Autodesk Inventor part; units mm, degrees
(part 3 of 3)
  arc A490 (-2990.6524, -2157.8219) -> (-2908.1943, -2279.9148) centre (-1432.224, -1194.1948) ccw
  arc A491 (-2908.1943, -2279.9148) -> (-2818.7411, -2390.8385) centre (-1616.1239, -1329.4704) ccw
  arc A492 (-2779.4113, -2436.604) -> (-2818.7411, -2390.8385) centre (-4535.4377, -3905.9087) ccw
  arc A493 (-2757.2128, -2466.1631) -> (-2779.4113, -2436.604) centre (-3049.0332, -2662.2024) ccw
  arc A494 (-2745.8364, -2486.6243) -> (-2757.2128, -2466.1631) centre (-2872.8883, -2543.8714) ccw
  arc A495 (-2745.9498, -2499.1945) -> (-2745.8364, -2486.6243) centre (-2759.5126, -2492.7865) ccw
  arc A496 (-2745.9498, -2499.1945) -> (-2749.3057, -2511.7301) centre (-2713.1452, -2514.6935) ccw
  arc A497 (-2749.3057, -2511.7301) -> (-2753.148, -2562.4823) centre (1336.3779, -2846.57) ccw
  arc A498 (-2753.148, -2562.4823) -> (-2756.6405, -2622.7286) centre (-124.1368, -2745.1096) ccw
  arc A499 (-2756.6405, -2622.7286) -> (-2759.272, -2690.9741) centre (1553.6701, -2823.1066) ccw
  line L62 (-2759.272, -2690.9741) -> (-2764.631, -2865.8991)
  line L63 (-2764.631, -2865.8991) -> (-2835.8911, -2780.9741)
  arc A500 (-2918.8006, -2674.4171) -> (-2835.8911, -2780.9741) centre (-1434.1321, -1604.7647) ccw
  arc A501 (-2986.2074, -2570.7172) -> (-2918.8006, -2674.4171) centre (-1871.837, -1920.1137) ccw
  arc A502 (-3041.5026, -2464.1872) -> (-2986.2074, -2570.7172) centre (-1942.3549, -1961.2823) ccw
  arc A503 (-3087.9821, -2349.1865) -> (-3041.5026, -2464.1872) centre (-1788.2283, -1890.7618) ccw
  arc A504 (-3121.0778, -2239.9227) -> (-3087.9821, -2349.1865) centre (-1890.4003, -1926.7975) ccw
  arc A505 (-3139.0551, -2142.0083) -> (-3121.0778, -2239.9227) centre (-2406.5893, -2058.1334) ccw
  arc A506 (-3147.4064, -2018.8391) -> (-3139.0551, -2142.0083) centre (-1814.454, -1990.3279) ccw
  arc A507 (-3149.631, -1810.813) -> (-3147.4064, -2018.8391) centre (6577.4997, -1810.8179) ccw
  line L64 (-3149.631, -1810.813) -> (-3149.631, -1522.7863)
  line L65 (-3149.631, -1522.7863) -> (-3120.6403, -1533.7291)
  arc A508 (-3120.6403, -1533.7291) -> (-3104.6551, -1538.5038) centre (-3078.921, -1423.2019) ccw
  arc A509 (-3104.6551, -1538.5038) -> (-3092.2345, -1539.1823) centre (-3096.4076, -1501.5506) ccw
  arc A510 (-3092.2345, -1539.1823) -> (-3080.2478, -1535.7989) centre (-3096.4218, -1501.4224) ccw
  arc A511 (-3080.2478, -1535.7989) -> (-3065.6403, -1527.6299) centre (-3131.0839, -1427.7506) ccw
  line L66 (-3065.6403, -1527.6299) -> (-3039.631, -1510.588)
  line L67 (-3039.631, -1510.588) -> (-3039.631, -70.8185)
  arc A512 (-3039.3783, 481.2624) -> (-3039.631, -70.8185) centre (599668.8589, -70.706) ccw
  arc A513 (-3038.5978, 946.0187) -> (-3039.3783, 481.2624) centre (301120.8498, 202.8683) ccw
  arc A514 (-3036.1137, 1368.9509) -> (-3037.5632, 1367.505) centre (-3036.1137, 1367.5015) ccw
  arc A515 (-3033.5939, 1368.2338) -> (-3036.1137, 1368.9509) centre (-3036.1137, 1364.1654) ccw
  arc A516 (-3013.7437, 1355.8898) -> (-3033.5939, 1368.2338) centre (-6444.9521, -4139.6549) ccw
  arc A517 (-2991.1032, 1341.5314) -> (-3013.7437, 1355.8898) centre (-4021.8968, -258.8014) ccw
  arc A518 (-2964.8997, 1324.4876) -> (-2991.1032, 1341.5314) centre (-4889.5902, -1605.9104) ccw
  arc A519 (3062.8013, -60.9811) -> (3061.4495, -1006.9802) centre (1295410.6067, -2380.7565) ccw
  arc A520 (3061.4495, -1006.9802) -> (3063.1224, -1310.9835) centre (26211.8445, -1031.5883) ccw
  arc A521 (3063.1224, -1310.9835) -> (3066.6099, -1479.2538) centre (12786.7982, -1193.6248) ccw
  arc A522 (3066.6099, -1479.2538) -> (3080.3013, -1510.9814) centre (3113.4039, -1477.8788) ccw
  arc A523 (3080.3013, -1510.9814) -> (3097.9046, -1523.8965) centre (3131.1382, -1460.1446) ccw
  arc A524 (3097.9046, -1523.8965) -> (3117.6763, -1530.0742) centre (3124.9899, -1471.939) ccw
  arc A525 (3117.6763, -1530.0742) -> (3138.8082, -1529.0661) centre (3125.3546, -1469.0395) ccw
  arc A526 (3138.8082, -1529.0661) -> (3160.3613, -1521.0532) centre (3120.1885, -1445.9896) ccw
  arc A527 (3170.8286, -1524.3232) -> (3160.3613, -1521.0532) centre (3163.9885, -1527.8306) ccw
  arc A528 (3176.5518, -1544.1089) -> (3170.8286, -1524.3232) centre (3122.861, -1548.9189) ccw
  arc A529 (3178.9628, -1593.2927) -> (3176.5518, -1544.1089) centre (2568.873, -1598.5484) ccw
  arc A530 (3179.8463, -1738.5532) -> (3178.9628, -1593.2927) centre (-25505.4744, -1840.3836) ccw
  arc A531 (3175.9829, -1976.8584) -> (3179.8463, -1738.5532) centre (-2851.4872, -1759.9572) ccw
  arc A532 (3160.8237, -2144.1805) -> (3175.9829, -1976.8584) centre (1631.4842, -1921.2765) ccw
  arc A533 (3130.6102, -2282.5675) -> (3160.8237, -2144.1805) centre (2161.9433, -1998.5905) ccw
  arc A534 (3079.9973, -2423.6115) -> (3130.6102, -2282.5675) centre (1918.6719, -1927.2727) ccw
  arc A535 (3039.5585, -2510.0751) -> (3079.9973, -2423.6115) centre (1772.8663, -1864.9587) ccw
  arc A536 (2995.4615, -2588.7548) -> (3039.5585, -2510.0751) centre (2029.2646, -1995.5405) ccw
  arc A537 (2943.0501, -2667.3464) -> (2995.4615, -2588.7548) centre (1922.5744, -1930.036) ccw
  arc A538 (2877.3135, -2753.7324) -> (2943.0501, -2667.3464) centre (1169.0771, -1385.6217) ccw
  line L68 (2877.3135, -2753.7324) -> (2795.369, -2856.0491)
  line L69 (2795.369, -2856.0491) -> (2789.4968, -2696.0491)
  arc A539 (2789.4968, -2696.0491) -> (2786.3804, -2632.67) centre (242.2861, -2789.5322) ccw
  arc A540 (2786.3804, -2632.67) -> (2781.8611, -2574.5881) centre (977.5322, -2744.1986) ccw
  arc A541 (2781.8611, -2574.5881) -> (2776.6989, -2526.2333) centre (864.468, -2754.8287) ccw
  arc A542 (2776.6989, -2526.2333) -> (2771.7488, -2507.2457) centre (2704.8711, -2534.82) ccw
  arc A543 (2767.4869, -2488.0525) -> (2771.7488, -2507.2457) centre (2824.6766, -2485.4232) ccw
  arc A544 (2771.2401, -2471.7334) -> (2767.4869, -2488.0525) centre (2798.6183, -2486.6212) ccw
  arc A545 (2786.0079, -2450.4453) -> (2771.2401, -2471.7334) centre (2876.4028, -2528.9192) ccw
  arc A546 (2829.1062, -2401.7678) -> (2786.0079, -2450.4453) centre (5301.222, -4633.9592) ccw
  arc A547 (2829.1062, -2401.7678) -> (2920.7467, -2290.528) centre (1649.3147, -1336.4763) ccw
  arc A548 (2920.7467, -2290.528) -> (3006.9234, -2165.8357) centre (1366.1527, -1123.9981) ccw
  arc A549 (3006.9234, -2165.8357) -> (3074.9751, -2050.5252) centre (1272.0921, -1064.2721) ccw
  arc A550 (3074.9751, -2050.5252) -> (3090.369, -1990.3095) centre (2964.9004, -1990.3095) ccw
  arc A551 (3090.369, -1990.3095) -> (3086.1599, -1969.8686) centre (3038.6292, -1990.3096) ccw
  arc A552 (3086.1599, -1969.8686) -> (3073.9361, -1950.2444) centre (3015.5336, -2000.2421) ccw
  arc A553 (3073.9361, -1950.2444) -> (3057.1368, -1935.9564) centre (3020.6955, -1995.8229) ccw
  arc A554 (3057.1368, -1935.9564) -> (3039.637, -1931.0491) centre (3039.637, -1964.7055) ccw
  arc A555 (3039.637, -1931.0491) -> (3014.6452, -1935.8643) centre (3039.637, -1998.3124) ccw
  arc A556 (3014.6452, -1935.8643) -> (2994.6509, -1949.5434) centre (3035.33, -1987.5505) ccw
  arc A557 (2994.6509, -1949.5434) -> (2973.9887, -1977.5702) centre (3104.4016, -2052.0851) ccw
  arc A558 (2973.9887, -1977.5702) -> (2943.1237, -2034.3477) centre (4298.6367, -2734.4439) ccw
  arc A559 (2902.337, -2106.6921) -> (2943.1237, -2034.3477) centre (1935.3983, -1513.8772) ccw
  arc A560 (2855.8027, -2176.9427) -> (2902.337, -2106.6921) centre (1877.629, -1478.4583) ccw
  arc A561 (2802.0044, -2247.2249) -> (2855.8027, -2176.9427) centre (1771.3658, -1402.5793) ccw
  arc A562 (2739.3728, -2319.6849) -> (2802.0044, -2247.2249) centre (1389.8938, -1089.9508) ccw
  line L70 (2739.3728, -2319.6849) -> (2683.3767, -2381.1337)
  line L71 (2683.3767, -2381.1337) -> (2632.1085, -2358.5914)
  line L72 (2632.1085, -2358.5914) -> (2580.8403, -2336.0491)
  line L73 (2580.8403, -2336.0491) -> (2580.6421, -711.0491)
  line L74 (2580.6421, -711.0491) -> (2580.4439, 913.9509)
  line L75 (2580.4439, 913.9509) -> (2623.3363, 931.5853)
  arc A563 (2623.3363, 931.5853) -> (2684.605, 968.0874) centre (2530.9143, 1156.3857) ccw
  arc A564 (2684.605, 968.0874) -> (2734.8197, 1021.8078) centre (2511.3163, 1180.3966) ccw
  arc A565 (2734.8197, 1021.8078) -> (2770.0399, 1088.4458) centre (2499.3492, 1188.8877) ccw
  arc A566 (2770.0399, 1088.4458) -> (2787.3675, 1162.7589) centre (2485.9178, 1193.8713) ccw
  arc A567 (2792.105, 1195.7029) -> (2787.3675, 1162.7589) centre (3201.5168, 1120.0149) ccw
  arc A568 (2799.1005, 1211.8828) -> (2792.105, 1195.7029) centre (2830.904, 1188.5302) ccw
  arc A569 (2812.8006, 1224.3388) -> (2799.1005, 1211.8828) centre (2836.7429, 1184.2428) ccw
  arc A570 (2846.3908, 1243.1416) -> (2812.8006, 1224.3388) centre (3165.391, 633.8599) ccw
  arc A571 (2846.3908, 1243.1416) -> (2872.3676, 1257.2794) centre (2420.1812, 2057.1904) ccw
  arc A572 (2872.3676, 1257.2794) -> (2907.0809, 1277.2085) centre (1391.313, 3877.2384) ccw
  arc A573 (2907.0809, 1277.2085) -> (2944.0271, 1299.0743) centre (1263.5319, 4096.4282) ccw
  arc A574 (2944.0271, 1299.0743) -> (2977.6923, 1319.6879) centre (1742.0091, 3299.9558) ccw
  arc A575 (3007.8259, 1338.2944) -> (2977.6923, 1319.6879) centre (4966.2802, -1867.1663) ccw
  arc A576 (3034.0202, 1354.0365) -> (3007.8259, 1338.2944) centre (4097.0708, -444.5093) ccw
  arc A577 (3056.8159, 1367.4393) -> (3034.0202, 1354.0365) centre (5954.021, -3586.2434) ccw
  arc A578 (3060.369, 1368.5548) -> (3056.8159, 1367.4393) centre (3061.0292, 1360.2354) ccw
  arc A579 (3062.4249, 1366.6589) -> (3060.369, 1368.5548) centre (3060.5197, 1366.6556) ccw
  arc A580 (3063.146, 948.7923) -> (3062.4249, 1366.6589) centre (-8702491.5883, -13865.3994) ccw
  arc A581 (3063.4266, 487.3009) -> (3063.146, 948.7923) centre (-207855.965, 589.788) ccw
  arc A582 (3062.8013, -60.9811) -> (3063.4266, 487.3009) centre (-414834.6536, 689.7528) ccw
  arc A583 (-1913.5687, 954.2396) -> (-1734.4782, 921.0323) centre (-866.4512, 6101.9309) ccw
  arc A584 (-1734.4782, 921.0323) -> (-1529.2527, 889.1161) centre (-270.2991, 9660.1238) ccw
  arc A585 (-1529.2527, 889.1161) -> (-1316.4625, 861.0585) centre (-198.9574, 10157.2039) ccw
  arc A586 (-1316.4625, 861.0585) -> (-1114.075, 839.4841) centre (-412.5654, 8380.3495) ccw
  arc A587 (-1114.075, 839.4841) -> (-975.393, 827.6361) centre (-258.4444, 10037.1738) ccw
  arc A588 (-975.393, 827.6361) -> (-837.5262, 817.9702) centre (-278.4862, 9779.7099) ccw
  arc A589 (-837.5262, 817.9702) -> (-657.2277, 807.634) centre (279.2554, 18720.7697) ccw
  arc A590 (-657.2277, 807.634) -> (-362.1635, 792.5791) centre (5502.6263, 118637.185) ccw
  line L76 (-362.1635, 792.5791) -> (-249.696, 786.982)
  line L77 (-249.696, 786.982) -> (-230.6402, 743.9032)
  arc A591 (-230.6402, 743.9032) -> (-205.8315, 701.8713) centre (-39.0236, 828.6645) ccw
  arc A592 (-205.8315, 701.8713) -> (-168.5998, 660.0881) centre (80.3764, 919.4226) ccw
  arc A593 (-168.5998, 660.0881) -> (-126.8329, 625.9013) centre (67.9455, 906.4746) ccw
  arc A594 (-126.8329, 625.9013) -> (-88.4851, 607.4261) centre (-49.6317, 737.1074) ccw
  line L78 (-88.4851, 607.4261) -> (-49.631, 595.7852)
  line L79 (-49.631, 595.7852) -> (-49.631, -1176.8374)
  line L80 (-49.631, -1176.8374) -> (-49.631, -2949.46)
  line L81 (-49.631, -2949.46) -> (-79.3693, -2955.9916)
  arc A595 (-79.3693, -2955.9916) -> (-115.6838, -2972.2525) centre (-58.3842, -3051.5361) ccw
  arc A596 (-115.6838, -2972.2525) -> (-160.8987, -3009.8378) centre (138.8628, -3324.4606) ccw
  arc A597 (-160.8987, -3009.8378) -> (-201.9746, -3054.7507) centre (144.5508, -3330.4312) ccw
  arc A598 (-201.9746, -3054.7507) -> (-226.1643, -3095.8525) centre (-68.3247, -3161.077) ccw
  line L82 (-226.1643, -3095.8525) -> (-244.631, -3140.541)
  line L83 (-244.631, -3140.541) -> (-349.631, -3135.1711)
  arc A599 (-882.8658, -3087.8365) -> (-349.631, -3135.1711) centre (15.6016, 4006.431) ccw
  arc A600 (-1366.8413, -3002.6041) -> (-882.8658, -3087.8365) centre (-244.0669, 1956.1506) ccw
  arc A601 (-1799.9599, -2880.1482) -> (-1366.8413, -3002.6041) centre (-426.4321, 1150.7475) ccw
  arc A602 (-2180.0572, -2720.7229) -> (-1799.9599, -2880.1482) centre (-832.1243, -39.841) ccw
  line L84 (-2180.0572, -2720.7229) -> (-2235.4834, -2692.8549)
  line L85 (-2235.4834, -2692.8549) -> (-2237.9929, -2610.9162)
  arc A603 (-2237.9929, -2610.9162) -> (-2240.3199, -2571.0685) centre (-2957.8229, -2632.9615) ccw
  arc A604 (-2240.3199, -2571.0685) -> (-2244.7516, -2538.0792) centre (-2589.6104, -2601.1989) ccw
  arc A605 (-2244.7516, -2538.0792) -> (-2251.5187, -2510.0686) centre (-2497.873, -2584.4084) ccw
  arc A606 (-2251.5187, -2510.0686) -> (-2260.9536, -2485.4694) centre (-2424.0386, -2562.1284) ccw
  arc A607 (-2260.9536, -2485.4694) -> (-2285.6695, -2445.4611) centre (-2448.0589, -2573.4192) ccw
  arc A608 (-2285.6695, -2445.4611) -> (-2322.761, -2404.7458) centre (-2588.4779, -2684.0657) ccw
  arc A609 (-2322.761, -2404.7458) -> (-2364.4619, -2370.44) centre (-2581.3125, -2676.5338) ccw
  arc A610 (-2364.4619, -2370.44) -> (-2403.1079, -2350.2383) centre (-2458.3199, -2502.9245) ccw
  line L86 (-2403.1079, -2350.2383) -> (-2439.631, -2337.0313)
  line L87 (-2439.631, -2337.0313) -> (-2439.5936, -711.5402)
  line L88 (-2439.5936, -711.5402) -> (-2439.5561, 913.9509)
  line L89 (-2439.5561, 913.9509) -> (-2396.4619, 931.6687)
  arc A611 (-2396.4619, 931.6687) -> (-2376.9013, 941.5424) centre (-2450.351, 1062.7406) ccw
  arc A612 (-2376.9013, 941.5424) -> (-2353.4806, 956.9654) centre (-2570.7261, 1261.3703) ccw
  arc A613 (-2353.4806, 956.9654) -> (-2330.1607, 974.9443) centre (-2585.0508, 1281.4419) ccw
  arc A614 (-2330.1607, 974.9443) -> (-2310.6579, 992.9047) centre (-2498.0086, 1176.7758) ccw
  line L90 (-2310.6579, 992.9047) -> (-2267.9481, 1036.4228)
  line L91 (-2267.9481, 1036.4228) -> (-2176.2896, 1012.7295)
  arc A615 (-2176.2896, 1012.7295) -> (-2129.5346, 1001.2725) centre (-1700.0863, 2854.9472) ccw
  arc A616 (-2129.5346, 1001.2725) -> (-2061.3062, 985.7746) centre (-293.3415, 8927.0311) ccw
  arc A617 (-2061.3062, 985.7746) -> (-1985.782, 969.299) centre (-96.1324, 9812.7982) ccw
  arc A618 (-1985.782, 969.299) -> (-1913.5687, 954.2396) centre (-418.6364, 8303.4593) ccw
  arc A619 (2330.7457, 994.7005) -> (2349.6048, 976.4208) centre (2502.3822, 1152.9096) ccw
  arc A620 (2349.6048, 976.4208) -> (2372.5893, 958.0878) centre (2588.9145, 1252.8727) ccw
  arc A621 (2372.5893, 958.0878) -> (2395.987, 942.3436) centre (2577.2368, 1236.9605) ccw
  arc A622 (2395.987, 942.3436) -> (2415.9142, 932.2005) centre (2468.6632, 1060.4771) ccw
  line L92 (2415.9142, 932.2005) -> (2460.294, 913.9509)
  line L93 (2460.294, 913.9509) -> (2460.3315, -712.7545)
  line L94 (2460.3315, -712.7545) -> (2460.369, -2339.46)
  line L95 (2460.369, -2339.46) -> (2430.6307, -2345.9916)
  arc A623 (2430.6307, -2345.9916) -> (2395.6917, -2361.6356) centre (2450.823, -2437.9267) ccw
  arc A624 (2395.6917, -2361.6356) -> (2350.0869, -2399.0009) centre (2680.5345, -2755.8033) ccw
  arc A625 (2350.0869, -2399.0009) -> (2307.6277, -2443.56) centre (2685.108, -2760.7414) ccw
  arc A626 (2307.6277, -2443.56) -> (2281.1542, -2484.427) centre (2458.3519, -2570.2071) ccw
  arc A627 (2281.1542, -2484.427) -> (2271.1872, -2509.3607) centre (2452.5649, -2567.4054) ccw
  arc A628 (2271.1872, -2509.3607) -> (2264.8592, -2535.3799) centre (2450.5721, -2566.7676) ccw
  arc A629 (2264.8592, -2535.3799) -> (2261.4364, -2566.4384) centre (2532.1364, -2580.5531) ccw
  arc A630 (2261.4364, -2566.4384) -> (2260.369, -2607.4076) centre (3047.127, -2607.4068) ccw
  line L96 (2260.369, -2607.4076) -> (2260.369, -2687.4517)
  line L97 (2260.369, -2687.4517) -> (2157.869, -2738.3674)
  arc A631 (1885.6632, -2855.5638) -> (2157.869, -2738.3674) centre (947.2098, -301.1524) ccw
  arc A632 (1576.3744, -2954.8591) -> (1885.6632, -2855.5638) centre (533.2985, 825.4938) ccw
  arc A633 (1238.9166, -3033.9584) -> (1576.3744, -2954.8591) centre (393.5214, 1332.1036) ccw
  arc A634 (881.9152, -3090.4282) -> (1238.9166, -3033.9584) centre (239.5431, 2127.3587) ccw
  arc A635 (774.7121, -3102.6312) -> (881.9152, -3090.4282) centre (161.6389, 2760.1604) ccw
  arc A636 (664.968, -3113.1563) -> (774.7121, -3102.6312) centre (106.361, 3288.8229) ccw
  arc A637 (534.0943, -3123.6818) -> (664.968, -3113.1563) centre (-176.4478, 6530.0766) ccw
  arc A638 (358.5435, -3136.0948) -> (534.0943, -3123.6818) centre (-1710.2072, 27368.8116) ccw
  line L98 (358.5435, -3136.0948) -> (271.7179, -3141.9829)
  line L99 (271.7179, -3141.9829) -> (252.0201, -3097.4527)
  arc A639 (252.0201, -3097.4527) -> (226.8939, -3054.645) centre (53.0153, -3185.4819) ccw
  arc A640 (226.8939, -3054.645) -> (189.6185, -3012.4784) centre (-58.6317, -3269.4916) ccw
  arc A641 (189.6185, -3012.4784) -> (147.8207, -2978.1362) centre (-44.7457, -3255.1153) ccw
  arc A642 (147.8207, -2978.1362) -> (109.223, -2959.5243) centre (70.1942, -3089.7909) ccw
  line L100 (109.223, -2959.5243) -> (70.369, -2947.8833)
  line L101 (70.369, -2947.8833) -> (70.369, -1180.6397)
  line L102 (70.369, -1180.6397) -> (70.369, 586.6039)
  line L103 (70.369, 586.6039) -> (124.685, 613.1783)
  arc A643 (124.685, 613.1783) -> (167.8117, 638.9579) centre (-7.2831, 882.9109) ccw
  arc A644 (167.8117, 638.9579) -> (205.1584, 671.1351) centre (5.4675, 865.1457) ccw
  arc A645 (205.1584, 671.1351) -> (235.1633, 708.2885) centre (17.9614, 853.0072) ccw
  arc A646 (235.1633, 708.2885) -> (256.4939, 748.8465) centre (50.7207, 831.1804) ccw
  line L104 (256.4939, 748.8465) -> (271.8098, 787.1245)
  line L105 (271.8098, 787.1245) -> (373.5894, 792.4972)
  arc A647 (427.4041, 795.2935) -> (373.5894, 792.4972) centre (2101.4454, -31940.1076) ccw
  arc A648 (511.565, 799.578) -> (427.4041, 795.2935) centre (9783.5496, -182160.9748) ccw
  arc A649 (606.7619, 804.3802) -> (511.565, 799.578) centre (10908.7538, -204363.8155) ccw
  arc A650 (700.369, 809.0576) -> (606.7619, 804.3802) centre (10238.2989, -191011.0651) ccw
  arc A651 (700.369, 809.0576) -> (1093.0397, 836.3644) centre (205.3886, 10763.7794) ccw
  arc A652 (1093.0397, 836.3644) -> (1472.2395, 878.5747) centre (309.3592, 9601.0173) ccw
  arc A653 (1472.2395, 878.5747) -> (1822.03, 933.4564) centre (458.966, 8478.8527) ccw
  arc A654 (1822.03, 933.4564) -> (2125.369, 999.0389) centre (1015.3399, 5398.953) ccw
  arc A655 (2183.3894, 1013.6184) -> (2125.369, 999.0389) centre (9876.5597, -29724.835) ccw
  arc A656 (2233.4491, 1026.0693) -> (2183.3894, 1013.6184) centre (6454.9688, -16053.7077) ccw
  arc A657 (2277.1003, 1036.8395) -> (2233.4491, 1026.0693) centre (15584.8039, -52992.3058) ccw
  arc A658 (2282.663, 1037.9163) -> (2277.1003, 1036.8395) centre (2290.577, 982.1241) ccw
  arc A659 (2287.1065, 1036.6495) -> (2282.663, 1037.9163) centre (2283.4612, 1032.2895) ccw
  arc A660 (2299.7961, 1025.6484) -> (2287.1065, 1036.6495) centre (1986.1488, 676.6788) ccw
  arc A661 (2314.5869, 1011.582) -> (2299.7961, 1025.6484) centre (2057.4823, 756.0457) ccw
  arc A662 (2330.7457, 994.7005) -> (2314.5869, 1011.582) centre (1874.0627, 573.7448) ccw
  arc A663 (2490.9409, -2639.684) -> (2505.8853, -2646.7865) centre (2551.8525, -2530.7929) ccw
  arc A664 (2505.8853, -2646.7865) -> (2517.1948, -2648.9704) centre (2517.3254, -2617.9183) ccw
  arc A665 (2517.1948, -2648.9704) -> (2529.0128, -2646.9546) centre (2517.3411, -2614.177) ccw
  arc A666 (2529.0128, -2646.9546) -> (2545.9409, -2639.9153) centre (2469.8448, -2480.7932) ccw
  arc A667 (2545.9409, -2639.9153) -> (2563.237, -2628.9559) centre (2508.6457, -2561.9285) ccw
  arc A668 (2563.237, -2628.9559) -> (2571.7932, -2616.5764) centre (2546.1929, -2608.0291) ccw
  arc A669 (2571.7932, -2616.5764) -> (2575.7925, -2595.8507) centre (2495.5121, -2591.1081) ccw
  arc A670 (2575.7925, -2595.8507) -> (2578.2797, -2543.0571) centre (364.474, -2465.2187) ccw
  line L106 (2578.2797, -2543.0571) -> (2581.1904, -2460.2721)
  line L107 (2581.1904, -2460.2721) -> (2609.6423, -2480.5316)
  arc A671 (2643.4506, -2519.1082) -> (2609.6423, -2480.5316) centre (2545.0501, -2571.243) ccw
  arc A672 (2661.2042, -2573.3624) -> (2643.4506, -2519.1082) centre (2495.2127, -2597.6479) ccw
  arc A673 (2668.8278, -2669.1243) -> (2661.2042, -2573.3624) centre (1938.7489, -2679.0613) ccw
  arc A674 (2670.369, -2895.6004) -> (2668.8278, -2669.1243) centre (-13973.0742, -2895.6158) ccw
  arc A675 (2669.6986, -3030.0281) -> (2670.369, -2895.6004) centre (-10804.9877, -2895.6124) ccw
  arc A676 (2667.5603, -3134.2249) -> (2669.6986, -3030.0281) centre (-2272.2812, -2980.7323) ccw
  arc A677 (2664.4733, -3214.9061) -> (2667.5603, -3134.2249) centre (-2952.3801, -2959.5989) ccw
  arc A678 (2659.7328, -3237.8981) -> (2664.4733, -3214.9061) centre (2589.9098, -3211.5171) ccw
  arc A679 (2617.088, -3299.3064) -> (2659.7328, -3237.8981) centre (2515.9908, -3183.5884) ccw
  arc A680 (2550.958, -3332.4809) -> (2617.088, -3299.3064) centre (2519.8906, -3188.0521) ccw
  arc A681 (2477.58, -3329.2633) -> (2550.958, -3332.4809) centre (2520.4231, -3190.527) ccw
  arc A682 (2414.8927, -3290.5645) -> (2477.58, -3329.2633) centre (2520.9094, -3188.9526) ccw
  line L108 (2414.8927, -3290.5645) -> (2385.369, -3259.761)
  line L109 (2385.369, -3259.761) -> (2382.3531, -2922.905)
  arc A683 (2381.6256, -2791.5061) -> (2382.3531, -2922.905) centre (21614.7948, -2750.7158) ccw
  arc A684 (2381.9551, -2675.5679) -> (2381.6256, -2791.5061) centre (14059.6173, -2766.7308) ccw
  arc A685 (2382.9678, -2577.1763) -> (2381.9551, -2675.5679) centre (22171.5681, -2830.0363) ccw
  arc A686 (2385.2333, -2553.9382) -> (2382.9678, -2577.1763) centre (2521.4308, -2578.9456) ccw
  arc A687 (2389.7676, -2539.3341) -> (2385.2333, -2553.9382) centre (2448.3349, -2565.5244) ccw
  arc A688 (2398.8325, -2521.8027) -> (2389.7676, -2539.3341) centre (2548.7354, -2610.4216) ccw
  arc A689 (2410.5199, -2504.3143) -> (2398.8325, -2521.8027) centre (2562.8614, -2618.7725) ccw
  arc A690 (2423.2491, -2489.6327) -> (2410.5199, -2504.3143) centre (2521.6666, -2587.8218) ccw
  line L110 (2423.2491, -2489.6327) -> (2455.369, -2457.4382)
  line L111 (2455.369, -2457.4382) -> (2460.369, -2541.4088)
  arc A691 (2460.369, -2541.4088) -> (2464.0505, -2591.6371) centre (4296.3427, -2432.0873) ccw
  arc A692 (2464.0505, -2591.6371) -> (2468.5613, -2614.5688) centre (2572.6845, -2582.1776) ccw
  arc A693 (2468.5613, -2614.5688) -> (2476.6105, -2628.4384) centre (2502.9909, -2603.8582) ccw
  arc A694 (2476.6105, -2628.4384) -> (2490.9409, -2639.684) centre (2519.6793, -2588.3087) ccw
  arc A695 (-2559.631, -2541.0491) -> (-2556.1243, -2591.8911) centre (-2189.3068, -2541.0489) ccw
  arc A696 (-2556.1243, -2591.8911) -> (-2544.5669, -2625.2727) centre (-2466.0956, -2579.4128) ccw
  arc A697 (-2544.5669, -2625.2727) -> (-2524.4099, -2644.1736) centre (-2502.6649, -2600.7846) ccw
  arc A698 (-2524.4099, -2644.1736) -> (-2495.3453, -2651.0491) centre (-2495.3453, -2586.1796) ccw
  arc A699 (-2495.3453, -2651.0491) -> (-2468.5276, -2645.1415) centre (-2495.3453, -2587.2255) ccw
  arc A700 (-2468.5276, -2645.1415) -> (-2451.346, -2628.8207) centre (-2484.071, -2611.5738) ccw
  arc A701 (-2451.346, -2628.8207) -> (-2442.1698, -2598.1342) centre (-2524.6584, -2590.1831) ccw
  arc A702 (-2442.1698, -2598.1342) -> (-2439.631, -2545.3348) centre (-2989.9362, -2545.3347) ccw
  arc A703 (-2439.3304, -2516.8507) -> (-2439.631, -2545.3348) centre (-1090.074, -2545.3353) ccw
  arc A704 (-2438.4025, -2492.8705) -> (-2439.3304, -2516.8507) centre (-1756.3445, -2531.2692) ccw
  arc A705 (-2437.1381, -2472.6263) -> (-2438.4025, -2492.8705) centre (-788.7023, -2585.7452) ccw
  arc A706 (-2435.4489, -2471.0491) -> (-2437.1381, -2472.6263) centre (-2435.4489, -2472.7423) ccw
  arc A707 (-2421.7438, -2474.1426) -> (-2435.4489, -2471.0491) centre (-2435.4489, -2502.9541) ccw
  arc A708 (-2407.1696, -2483.4129) -> (-2421.7438, -2474.1426) centre (-2452.0989, -2537.9566) ccw
  arc A709 (-2392.4689, -2498.2276) -> (-2407.1696, -2483.4129) centre (-2473.4852, -2563.9193) ccw
  arc A710 (-2378.3986, -2518.0432) -> (-2392.4689, -2498.2276) centre (-2540.3421, -2618.1299) ccw
  arc A711 (-2365.6773, -2549.7478) -> (-2378.3986, -2518.0432) centre (-2463.2936, -2570.5112) ccw
  arc A712 (-2359.5831, -2594.8277) -> (-2365.6773, -2549.7478) centre (-2661.7641, -2612.7269) ccw
  arc A713 (-2356.9187, -2676.1973) -> (-2359.5831, -2594.8277) centre (-3897.0904, -2685.9011) ccw
  arc A714 (-2355.9702, -2896.6847) -> (-2356.9187, -2676.1973) centre (-57478.2393, -3023.5607) ccw
  arc A715 (-2355.9023, -3114.6567) -> (-2355.9702, -2896.6847) centre (-57122.7363, -3022.736) ccw
  arc A716 (-2358.1209, -3196.2776) -> (-2355.9023, -3114.6567) centre (-3957.2868, -3111.9689) ccw
  arc A717 (-2363.5782, -3240.5905) -> (-2358.1209, -3196.2776) centre (-2677.463, -3179.4418) ccw
  arc A718 (-2375.5229, -3267.5648) -> (-2363.5782, -3240.5905) centre (-2428.625, -3227.9185) ccw
  arc A719 (-2420.1174, -3310.9015) -> (-2375.5229, -3267.5648) centre (-2533.4901, -3149.6255) ccw
  arc A720 (-2472.7912, -3334.0725) -> (-2420.1174, -3310.9015) centre (-2504.1106, -3191.4189) ccw
  arc A721 (-2527.5239, -3334.2954) -> (-2472.7912, -3334.0725) centre (-2500.6753, -3207.0654) ccw
  arc A722 (-2578.2062, -3312.0637) -> (-2527.5239, -3334.2954) centre (-2499.5103, -3201.5454) ccw
  arc A723 (-2614.7179, -3273.3349) -> (-2578.2062, -3312.0637) centre (-2498.9731, -3200.7912) ccw
  arc A724 (-2632.4142, -3224.6064) -> (-2614.7179, -3273.3349) centre (-2510.097, -3207.763) ccw
  arc A725 (-2638.4633, -3136.7644) -> (-2632.4142, -3224.6064) centre (-1991.3896, -3136.3344) ccw
  arc A726 (-2637.4995, -2881.478) -> (-2638.4633, -3136.7644) centre (26110.3522, -3117.6544) ccw
  line L112 (-2637.4995, -2881.478) -> (-2634.631, -2532.3388)
  line L113 (-2634.631, -2532.3388) -> (-2605.2601, -2501.6939)
  arc A727 (-2593.4176, -2489.9562) -> (-2605.2601, -2501.6939) centre (-2370.7309, -2726.4733) ccw
  arc A728 (-2582.129, -2480.051) -> (-2593.4176, -2489.9562) centre (-2446.637, -2645.8523) ccw
  arc A729 (-2572.3928, -2472.5521) -> (-2582.129, -2480.051) centre (-2447.2621, -2645.087) ccw
  arc A730 (-2567.7601, -2471.0491) -> (-2572.3928, -2472.5521) centre (-2567.7601, -2478.9398) ccw
  arc A731 (-2564.5352, -2473.782) -> (-2567.7601, -2471.0491) centre (-2567.7601, -2474.3183) ccw
  arc A732 (-2562.019, -2491.6116) -> (-2564.5352, -2473.782) centre (-2925.7591, -2533.8525) ccw
  arc A733 (-2560.2161, -2514.2109) -> (-2562.019, -2491.6116) centre (-2874.7907, -2527.9338) ccw
  arc A734 (-2559.631, -2541.0491) -> (-2560.2161, -2514.2109) centre (-3175.4615, -2541.0496) ccw
  arc A735 (-2160.3969, -2860.6625) -> (-1826.0099, -2999.0036) centre (-1075.1723, -710.8422) ccw
  arc A736 (-1826.0099, -2999.0036) -> (-1411.0361, -3114.8346) centre (-328.6054, 1564.3139) ccw
  arc A737 (-1411.0361, -3114.8346) -> (-955.023, -3200.082) centre (-181.2792, 2201.1929) ccw
  arc A738 (-955.023, -3200.082) -> (-494.631, -3246.0049) centre (-189.492, 2143.8674) ccw
  arc A739 (-451.0443, -3248.5774) -> (-494.631, -3246.0049) centre (-1008.7806, -12327.8468) ccw
  arc A740 (-402.7092, -3251.632) -> (-451.0443, -3248.5774) centre (-1294.6459, -16981.6679) ccw
  arc A741 (-356.9623, -3254.6854) -> (-402.7092, -3251.632) centre (-1238.5218, -16117.8448) ccw
  arc A742 (-322.131, -3257.2109) -> (-356.9623, -3254.6854) centre (-659.0558, -7662.7212) ccw
  line L114 (-322.131, -3257.2109) -> (-249.631, -3262.7555)
  line L115 (-249.631, -3262.7555) -> (-249.631, -3497.1362)
  line L116 (-249.631, -3497.1362) -> (-249.631, -3731.517)
  line L117 (-249.631, -3731.517) -> (-332.131, -3725.9456)
  arc A743 (-866.7594, -3673.8575) -> (-332.131, -3725.9456) centre (277.4429, 5300.4099) ccw
  arc A744 (-1318.03, -3594.334) -> (-866.7594, -3673.8575) centre (-257.9931, 1100.8672) ccw
  arc A745 (-1716.7667, -3481.5073) -> (-1318.03, -3594.334) centre (-467.98, 170.7908) ccw
  arc A746 (-2091.1559, -3328.8116) -> (-1716.7667, -3481.5073) centre (-584.5335, -170.1011) ccw
  line L118 (-2091.1559, -3328.8116) -> (-2237.6807, -3258.9229)
  line L119 (-2237.6807, -3258.9229) -> (-2238.7185, -3182.486)
  arc A747 (-2238.0305, -3095.8943) -> (-2238.7185, -3182.486) centre (-226.9057, -3155.1708) ccw
  arc A748 (-2233.4246, -2971.4332) -> (-2238.0305, -3095.8943) centre (6035.0937, -3339.7393) ccw
  arc A749 (-2227.2322, -2835.0289) -> (-2233.4246, -2971.4332) centre (77819.1465, -6537.2973) ccw
  arc A750 (-2223.064, -2831.0491) -> (-2227.2322, -2835.0289) centre (-2223.064, -2835.2217) ccw
  arc A751 (-2220.1835, -2831.6872) -> (-2223.064, -2831.0491) centre (-2223.064, -2837.87) ccw
  arc A752 (-2203.0042, -2839.748) -> (-2220.1835, -2831.6872) centre (-3689.0196, -5984.4086) ccw
  arc A753 (-2183.1702, -2849.3127) -> (-2203.0042, -2839.748) centre (-2799.3569, -4101.735) ccw
  arc A754 (-2160.3969, -2860.6625) -> (-2183.1702, -2849.3127) centre (-3278.426, -5075.4615) ccw
  line L120 (2259.9611, -3044.6266) -> (2259.1952, -3258.2041)
  line L121 (2259.1952, -3258.2041) -> (2122.2821, -3324.3349)
  arc A755 (1768.9741, -3469.3543) -> (2122.2821, -3324.3349) centre (748.0582, -479.2292) ccw
  arc A756 (1367.2701, -3586.1449) -> (1768.9741, -3469.3543) centre (301.8107, 827.7576) ccw
  arc A757 (937.666, -3669.9179) -> (1367.2701, -3586.1449) centre (206.9864, 1220.5859) ccw
  arc A758 (500.369, -3715.8443) -> (937.666, -3669.9179) centre (193.5294, 1310.6498) ccw
  arc A759 (500.369, -3715.8443) -> (459.4211, -3718.4669) centre (918.1678, -10560.0263) ccw
  arc A760 (459.4211, -3718.4669) -> (414.9158, -3721.5553) centre (1100.4687, -13278.6966) ccw
  arc A761 (414.9158, -3721.5553) -> (373.4496, -3724.6279) centre (1046.822, -12530.6813) ccw
  arc A762 (373.4496, -3724.6279) -> (342.869, -3727.1422) centre (578.0202, -6399.9346) ccw
  line L122 (342.869, -3727.1422) -> (280.369, -3732.6409)
  line L123 (280.369, -3732.6409) -> (280.369, -3497.6409)
  line L124 (280.369, -3497.6409) -> (280.369, -3262.6409)
  line L125 (280.369, -3262.6409) -> (342.869, -3257.1667)
  arc A763 (374.3545, -3254.6697) -> (342.869, -3257.1667) centre (510.3804, -5169.6647) ccw
  arc A764 (419.3221, -3251.6084) -> (374.3545, -3254.6697) centre (917.831, -10905.8846) ccw
  arc A765 (468.6728, -3248.5387) -> (419.3221, -3251.6084) centre (970.7087, -11717.9193) ccw
  arc A766 (515.369, -3245.9321) -> (468.6728, -3248.5387) centre (870.446, -10026.5663) ccw
  arc A767 (515.369, -3245.9321) -> (790.5395, -3223.0426) centre (279.9574, 1249.5688) ccw
  arc A768 (790.5395, -3223.0426) -> (1086.5602, -3181.9687) centre (90.3914, 2910.2026) ccw
  arc A769 (1086.5602, -3181.9687) -> (1378.2811, -3126.9522) centre (101.6777, 2841.2162) ccw
  arc A770 (1378.2811, -3126.9522) -> (1640.369, -3061.9773) centre (503.4725, 962.8222) ccw
  arc A771 (1640.369, -3061.9773) -> (1785.3152, -3017.1681) centre (799.4738, -85.0662) ccw
  arc A772 (1785.3152, -3017.1681) -> (1944.3765, -2960.5147) centre (274.8353, 1475.3065) ccw
  arc A773 (1944.3765, -2960.5147) -> (2091.5108, -2902.118) centre (382.1285, 1190.2276) ccw
  arc A774 (2091.5108, -2902.118) -> (2195.369, -2853.0875) centre (1603.8066, -1734.5315) ccw
  arc A775 (2211.613, -2844.9558) -> (2195.369, -2853.0875) centre (2385.4009, -3212.4102) ccw
  arc A776 (2227.3434, -2838.0173) -> (2211.613, -2844.9558) centre (2351.0865, -3139.8567) ccw
  arc A777 (2240.8457, -2832.8596) -> (2227.3434, -2838.0173) centre (2340.7234, -3114.5774) ccw
  arc A778 (2248.048, -2831.491) -> (2240.8457, -2832.8596) centre (2248.8862, -2855.539) ccw
  arc A779 (2254.7832, -2837.3226) -> (2248.048, -2831.491) centre (2248.276, -2838.0329) ccw
  arc A780 (2257.9333, -2875.5207) -> (2254.7832, -2837.3226) centre (1534.2401, -2915.9716) ccw
  arc A781 (2259.816, -2936.1384) -> (2257.9333, -2875.5207) centre (1036.3402, -2943.8001) ccw
  arc A782 (2259.9611, -3044.6266) -> (2259.816, -2936.1384) centre (-8756.315, -3005.1204) ccw
  arc A783 (-25.2197, -3246.8832) -> (-6.8775, -3257.0782) centre (25.1412, -3177.8742) ccw
  arc A784 (-6.8775, -3257.0782) -> (10.5294, -3260.2913) centre (9.6856, -3216.1064) ccw
  arc A785 (10.5294, -3260.2913) -> (28.3908, -3256.46) centre (9.6163, -3212.484) ccw
  arc A786 (28.3908, -3256.46) -> (48.1439, -3245.482) centre (-14.4452, -3156.1236) ccw
  arc A787 (48.1439, -3245.482) -> (60.1171, -3233.6884) centre (19.1125, -3204.0338) ccw
  arc A788 (60.1171, -3233.6884) -> (66.683, -3219.2847) centre (27.5824, -3210.1593) ccw
  arc A789 (66.683, -3219.2847) -> (69.6704, -3196.3943) centre (-46.4685, -3192.8771) ccw
  arc A790 (69.6704, -3196.3943) -> (70.369, -3150.2515) centre (-1453.9645, -3150.2511) ccw
  line L126 (70.369, -3150.2515) -> (70.369, -3070.588)
  line L127 (70.369, -3070.588) -> (95.8801, -3087.3035)
  arc A791 (129.4577, -3121.8846) -> (95.8801, -3087.3035) centre (35.3771, -3179.6429) ccw
  arc A792 (146.8556, -3168.9259) -> (129.4577, -3121.8846) centre (19.9123, -3189.1372) ccw
  arc A793 (154.4122, -3253.7427) -> (146.8556, -3168.9259) centre (-462.732, -3265.9809) ccw
  arc A794 (157.5159, -3474.4276) -> (154.4122, -3253.7427) centre (-18987.26, -3633.3135) ccw
  arc A795 (157.8177, -3595.5867) -> (157.5159, -3474.4276) centre (-10276.2024, -3561.0042) ccw
  arc A796 (156.5865, -3704.4463) -> (157.8177, -3595.5867) centre (-6651.5169, -3573.0093) ccw
  arc A797 (154.353, -3795.7986) -> (156.5865, -3704.4463) centre (-8727.4256, -3532.935) ccw
  arc A798 (150.7586, -3824.4276) -> (154.353, -3795.7986) centre (2.8214, -3791.314) ccw
  arc A799 (135.3121, -3862.7953) -> (150.7586, -3824.4276) centre (26.0476, -3796.5131) ccw
  arc A800 (107.6476, -3896.8824) -> (135.3121, -3862.7953) centre (-2.6143, -3779.1262) ccw
  arc A801 (71.6374, -3922.4191) -> (107.6476, -3896.8824) centre (-3.8706, -3777.7844) ccw
  arc A802 (31.8106, -3935.8055) -> (71.6374, -3922.4191) centre (9.4114, -3803.2259) ccw
  arc A803 (-7.1977, -3936.3246) -> (31.8106, -3935.8055) centre (10.635, -3810.4676) ccw
  arc A804 (-45.425, -3925.1001) -> (-7.1977, -3936.3246) centre (12.164, -3799.6765) ccw
  arc A805 (-79.6606, -3903.0726) -> (-45.425, -3925.1001) centre (14.8903, -3793.7388) ccw
  arc A806 (-106.9991, -3872.0702) -> (-79.6606, -3903.0726) centre (20.713, -3787.0061) ccw
  arc A807 (-120.3927, -3841.4421) -> (-106.9991, -3872.0702) centre (-27.2542, -3818.9552) ccw
  arc A808 (-126.7059, -3799.4598) -> (-120.3927, -3841.4421) centre (115.342, -3784.5274) ccw
  arc A809 (-129.2069, -3723.1296) -> (-126.7059, -3799.4598) centre (1194.0993, -3717.9767) ccw
  arc A810 (-129.631, -3505.2212) -> (-129.2069, -3723.1296) centre (55859.3153, -3505.193) ccw
  arc A811 (-128.9569, -3369.8781) -> (-129.631, -3505.2212) centre (13459.2935, -3505.2299) ccw
  arc A812 (-126.8612, -3258.2152) -> (-128.9569, -3369.8781) centre (6212.1282, -3433.041) ccw
  arc A813 (-123.9267, -3167.0017) -> (-126.8612, -3258.2152) centre (9810.6594, -3532.2691) ccw
  arc A814 (-119.7329, -3146.317) -> (-123.9267, -3167.0017) centre (-59.0548, -3169.3868) ccw
  arc A815 (-113.9873, -3134.5117) -> (-119.7329, -3146.317) centre (-51.1796, -3172.3808) ccw
  arc A816 (-104.6343, -3120.3931) -> (-113.9873, -3134.5117) centre (56.6534, -3237.397) ccw
  arc A817 (-93.5265, -3106.3534) -> (-104.6343, -3120.3931) centre (69.002, -3246.3551) ccw
  arc A818 (-82.2329, -3094.6239) -> (-93.5265, -3106.3534) centre (17.8859, -3202.3238) ccw
  line L128 (-82.2329, -3094.6239) -> (-54.631, -3068.9649)
  line L129 (-54.631, -3068.9649) -> (-49.631, -3150.8411)
  arc A819 (-49.631, -3150.8411) -> (-46.2272, -3193.8037) centre (1140.6259, -3078.1551) ccw
  arc A820 (-46.2272, -3193.8037) -> (-41.7731, -3219.2896) centre (123.6048, -3177.2551) ccw
  arc A821 (-41.7731, -3219.2896) -> (-35.194, -3235.6801) centre (22.8607, -3202.8615) ccw
  arc A822 (-35.194, -3235.6801) -> (-25.2197, -3246.8832) centre (-4.2981, -3218.2145) ccw
  arc A823 (-409.631, 2773.0271) -> (-1144.387, 2723.0887) centre (105.5536, -10237.323) ccw
  arc A824 (-1144.387, 2723.0887) -> (-1813.6535, 2633.6758) centre (-260.2742, -6444.0816) ccw
  arc A825 (-1813.6535, 2633.6758) -> (-2384.7101, 2511.7433) centre (-608.8226, -4407.2117) ccw
  arc A826 (-2384.7101, 2511.7433) -> (-2813.2484, 2361.722) centre (-1723.7785, -63.2918) ccw
  arc A827 (-2813.2484, 2361.722) -> (-2879.3621, 2330.5307) centre (-2007.0004, 567.116) ccw
  arc A828 (-2879.3621, 2330.5307) -> (-2919.5448, 2307.1654) centre (-2726.0958, 2020.7143) ccw
  arc A829 (-2919.5448, 2307.1654) -> (-2942.5295, 2287.5765) centre (-2843.817, 2195.0311) ccw
  arc A830 (-2942.5295, 2287.5765) -> (-2949.631, 2269.6186) centre (-2923.3748, 2269.6186) ccw
  arc A831 (-2949.631, 2269.6186) -> (-2944.8137, 2250.4223) centre (-2908.9754, 2269.6186) ccw
  arc A832 (-2944.8137, 2250.4223) -> (-2928.9413, 2225.8565) centre (-2787.228, 2334.8305) ccw
  arc A833 (-2928.9413, 2225.8565) -> (-2909.9263, 2204.7818) centre (-2785.5298, 2336.1362) ccw
  arc A834 (-2909.9263, 2204.7818) -> (-2895.2895, 2198.9509) centre (-2895.2895, 2220.2373) ccw
  arc A835 (-2895.2895, 2198.9509) -> (-2886.8448, 2200.5112) centre (-2895.2895, 2222.5835) ccw
  arc A836 (-2886.8448, 2200.5112) -> (-2861.545, 2210.4802) centre (-3375.3402, 3477.3263) ccw
  arc A837 (-2861.545, 2210.4802) -> (-2831.5875, 2223.1644) centre (-3263.1825, 3200.7845) ccw
  arc A838 (-2831.5875, 2223.1644) -> (-2798.5153, 2238.1996) centre (-3501.8205, 3741.3343) ccw
  arc A839 (-2310.7202, 2407.8227) -> (-2798.5153, 2238.1996) centre (-1733.9336, -37.0794) ccw
  arc A840 (-1617.2332, 2541.3101) -> (-2310.7202, 2407.8227) centre (-357.2399, -5872.6719) ccw
  arc A841 (-818.0426, 2629.4137) -> (-1617.2332, 2541.3101) centre (-84.229, -7695.8216) ccw
  arc A842 (10.369, 2658.8297) -> (-818.0426, 2629.4137) centre (10.8093, -9033.136) ccw
  arc A843 (835.2983, 2629.7074) -> (10.369, 2658.8297) centre (10.8158, -9026.7184) ccw
  arc A844 (1632.7209, 2542.3649) -> (835.2983, 2629.7074) centre (99.6998, -7770.0321) ccw
  arc A845 (2324.8194, 2410.2544) -> (1632.7209, 2542.3649) centre (369.9927, -5951.7282) ccw
  arc A846 (2809.3297, 2242.739) -> (2324.8194, 2410.2544) centre (1758.5436, -12.044) ccw
  arc A847 (2809.3297, 2242.739) -> (2846.3103, 2225.9641) centre (3646.4063, 4038.9397) ccw
  arc A848 (2846.3103, 2225.9641) -> (2879.6666, 2211.8137) centre (3354.2977, 3377.0351) ccw
  arc A849 (2879.6666, 2211.8137) -> (2907.8668, 2200.6225) centre (3513.8333, 3768.6979) ccw
  arc A850 (2907.8668, 2200.6225) -> (2916.8297, 2198.9509) centre (2916.8297, 2223.8161) ccw
  arc A851 (2916.8297, 2198.9509) -> (2933.6311, 2204.3633) centre (2916.8297, 2227.7352) ccw
  arc A852 (2933.6311, 2204.3633) -> (2951.6972, 2221.0791) centre (2875.2326, 2285.6) ccw
  arc A853 (2951.6972, 2221.0791) -> (2965.714, 2242.4757) centre (2870.6766, 2289.4445) ccw
  arc A854 (2965.714, 2242.4757) -> (2970.369, 2262.4011) centre (2925.3969, 2262.401) ccw
  arc A855 (2970.369, 2262.4011) -> (2962.9227, 2286.8164) centre (2926.6186, 2262.401) ccw
  arc A856 (2962.9227, 2286.8164) -> (2941.7548, 2308.3635) centre (2894.601, 2240.8683) ccw
  arc A857 (2941.7548, 2308.3635) -> (2900.007, 2332.3522) centre (2785.3336, 2084.4641) ccw
  arc A858 (2900.007, 2332.3522) -> (2818.6412, 2368.4017) centre (1748.1302, -157.6516) ccw
  arc A859 (2818.6412, 2368.4017) -> (2434.8711, 2502.1324) centre (1607.9412, -488.4497) ccw
  arc A860 (2434.8711, 2502.1324) -> (1970.1566, 2610.4872) centre (872.1215, -3149.5066) ccw
  arc A861 (1970.1566, 2610.4872) -> (1425.0366, 2694.5791) centre (507.5398, -5061.9353) ccw
  arc A862 (1425.0366, 2694.5791) -> (795.369, 2754.1028) centre (-156.6239, -10676.6965) ccw
  arc A863 (795.369, 2754.1028) -> (582.0952, 2764.2654) centre (469.2662, -1846.5441) ccw
  arc A864 (582.0952, 2764.2654) -> (192.6934, 2772.0875) centre (-505.1288, -41663.5785) ccw
  arc A865 (192.6934, 2772.0875) -> (-196.7395, 2776.4998) centre (-506.3919, -41742.2824) ccw
  arc A866 (-196.7395, 2776.4998) -> (-409.631, 2773.0271) centre (-228.5708, -1799.389) ccw
  line L130 (-240.3697, 3101.0693) -> (-225.9643, 3145.3268)
  point P0 (0, 0)
  point P1 (17558894.8355, -41953.2381)
  point P2 (-3037.5632, 1367.505)
  point P3 (-3038.5978, 946.0187)
  constraints: 1735 point on circle, 867 centre point, 262 end point, 4 other
ref_plane "Work Plane1" through (0, 0, 152.4) normal (0, 0, 1) x (1, 0, 0)
sketch "Sketch16" plane through (0, 0, 304.8) normal (0, 0, 1) x (1, 0, 0)
  line L0 (-1485.6663, 2267.6369) -> (-1176.5052, 1752.3685)
  line L1 (-1176.5052, 1752.3685) -> (-477.2124, 2171.9442)
  line L2 (-477.2124, 2171.9442) -> (-477.2124, -1972.2862)
  line L3 (-477.2124, -1972.2862) -> (-1927.3249, -1972.2862)
  line L4 (-1927.3249, -1972.2862) -> (-1927.3249, -2885.0474)
  line L5 (-1927.3249, -2885.0474) -> (1605.9442, -2885.0474)
  line L6 (1605.9442, -2885.0474) -> (1605.9442, -1972.2862)
  line L7 (1605.9442, -1972.2862) -> (250.2732, -1972.2862)
  line L8 (250.2732, -1972.2862) -> (250.2732, 2608.4355)
  line L9 (250.2732, 2608.4355) -> (250.2732, 3309.2006)
  line L10 (250.2732, 3309.2006) -> (-1485.6663, 2267.6369)
  point P0 (0, 0)
  constraints: 22 end point, 6 perpendicular, 3 vertical, 1 point on line
extrude "Extrusion7" add sketch "Sketch16" along normal blind 127
body "Solid1"
